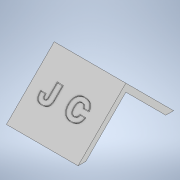
# Autodesk Inventor part: Tablero
Saved by Autodesk Inventor 2022 (Build 260153000, 153)
## iProperties
Created: 2022-08-27
Part Number: Tablero
Material: Generic
Document SubType Name: Modeling
Designer: Wulics
Density: 1 g/cm^3
Appearance: Default
Author: Wulics
Autodesk Inventor part; units mm, degrees
note: some values were not read from the file. Chosen so that the rebuilt part matches the saved one: direction of "Emboss1".
ref_plane "YZ Plane" through (0, 0, 0) normal (1, 0, 0) x (0, 1, 0)
ref_plane "XZ Plane" through (0, 0, 0) normal (0, 1, 0) x (-1, 0, 0)
ref_plane "XY Plane" through (0, 0, 0) normal (0, 0, 1) x (1, 0, 0)
sketch "Sketch1" plane through (0, 0, 0) normal (1, 0, 0) x (0, 1, 0)
  line L0 (0, 0) -> (173.2412, -173.2412)
  line L1 (173.2412, -173.2412) -> (0, -346.4823)
  line L2 (0, -346.4823) -> (0, -318.1981)
  line L3 (0, -318.1981) -> (144.9569, -173.2412)
  line L4 (144.9569, -173.2412) -> (0, -28.2843)
  line L5 (0, -28.2843) -> (0, 0)
  dimension "d0" = 245
  dimension "d1" = 245
  dimension "d2" = 90
  dimension "d3" = 20
  dimension "d4" = 20
  constraints: 12 end point, 2 parallel, 1 collinear, 1 point on line, 1 vertical
  measures "d0" distance of L0.start L0.end
  measures "d1" distance of L0.end L1.end
  measures "d2" angle of L3 L4
  measures "d3" distance between parallel lines of L0 L4
  measures "d4" distance between parallel lines of L1 L3
extrude "Extrusion1" add sketch "Sketch1" along normal blind 260
sketch "Sketch2" plane through (0, 0, 0) normal (0, 0.7071068, 0.7071068) x (1, 0, 0)
  line L0 (37.9204, 161.6588) -> (217.6406, 161.6588) construction
  line L1 (217.6406, 161.6588) -> (217.6406, 17.7751) construction
  line L2 (217.6406, 17.7751) -> (37.9204, 17.7751) construction
  line L3 (37.9204, 17.7751) -> (37.9204, 161.6588) construction
  line L4 (39.9742, 120.0125) -> (59.8275, 120.0125)
  line L5 (59.8275, 120.0125) -> (59.8275, 113.5088)
  spline S0 degree 2 poles (59.8275, 113.5088) (59.8275, 109.173) (62.5088, 105.6359) (65.5895, 105.6359) knots 0 0 0 1 2 2 2
  spline S1 degree 2 poles (65.5895, 105.6359) (68.8413, 105.6359) (71.5227, 109.4583) (71.5227, 115.0492) knots 0 0 0 1 2 2 2
  line L6 (71.5227, 115.0492) -> (71.5227, 159.8332)
  line L7 (71.5227, 159.8332) -> (94.0003, 159.8332)
  line L8 (94.0003, 159.8332) -> (94.0003, 112.7101)
  spline S2 degree 2 poles (94.0003, 112.7101) (94.0003, 100.5585) (79.909, 87.8935) (66.3312, 87.8935) knots 0 0 0 1 2 2 2
  spline S3 degree 2 poles (66.3312, 87.8935) (52.6392, 87.8935) (39.9742, 101.4143) (39.9742, 116.1331) knots 0 0 0 1 2 2 2
  line L9 (39.9742, 116.1331) -> (39.9742, 120.0125)
  line L10 (57.4314, 111.6832) -> (57.4314, 117.7875)
  line L11 (57.4314, 117.7875) -> (42.4844, 117.7875)
  line L12 (42.4844, 117.7875) -> (42.4844, 114.9351)
  spline S4 degree 2 poles (42.4844, 114.9351) (42.4844, 102.213) (54.3507, 90.1184) (66.8446, 90.1184) knots 0 0 0 1 2 2 2
  spline S5 degree 2 poles (66.8446, 90.1184) (79.3385, 90.1184) (91.5471, 102.27) (91.5471, 114.6498) knots 0 0 0 1 2 2 2
  line L13 (91.5471, 114.6498) -> (91.5471, 157.4371)
  line L14 (91.5471, 157.4371) -> (73.9188, 157.4371)
  line L15 (73.9188, 157.4371) -> (73.9188, 113.3377)
  spline S6 degree 2 poles (73.9188, 113.3377) (73.9188, 108.032) (69.8682, 103.411) (65.2472, 103.411) knots 0 0 0 1 2 2 2
  spline S7 degree 2 poles (65.2472, 103.411) (61.539, 103.411) (57.4314, 107.7468) (57.4314, 111.6832) knots 0 0 0 1 2 2 2
  line L16 (184.31, 116.9888) -> (205.5895, 116.9888)
  spline S8 degree 2 poles (205.5895, 116.9888) (204.7338, 103.2399) (187.0483, 87.8935) (172.0443, 87.8935) knots 0 0 0 1 2 2 2
  spline S9 degree 2 poles (172.0443, 87.8935) (155.2146, 87.8935) (135.9318, 107.6327) (135.9318, 124.8047) knots 0 0 0 1 2 2 2
  spline S10 degree 2 poles (135.9318, 124.8047) (135.9318, 141.8625) (155.0435, 161.6588) (171.5308, 161.6588) knots 0 0 0 1 2 2 2
  spline S11 degree 2 poles (171.5308, 161.6588) (186.706, 161.6588) (204.2203, 146.9399) (205.1902, 133.3621) knots 0 0 0 1 2 2 2
  line L17 (205.1902, 133.3621) -> (183.6824, 133.3621)
  spline S12 degree 2 poles (183.6824, 133.3621) (183.226, 138.7248) (177.2358, 144.1445) (171.8161, 144.1445) knots 0 0 0 1 2 2 2
  spline S13 degree 2 poles (171.8161, 144.1445) (165.1983, 144.1445) (158.5805, 134.5031) (158.5805, 124.7476) knots 0 0 0 1 2 2 2
  spline S14 degree 2 poles (158.5805, 124.7476) (158.5805, 115.2203) (165.5977, 105.4077) (172.4436, 105.4077) knots 0 0 0 1 2 2 2
  spline S15 degree 2 poles (172.4436, 105.4077) (177.5781, 105.4077) (183.7965, 111.455) (184.31, 116.9888) knots 0 0 0 1 2 2 2
  line L18 (202.9082, 114.7639) -> (186.4208, 114.7639)
  spline S16 degree 2 poles (186.4208, 114.7639) (185.7362, 109.5153) (178.0345, 103.2399) (172.3295, 103.2399) knots 0 0 0 1 2 2 2
  spline S17 degree 2 poles (172.3295, 103.2399) (164.4567, 103.2399) (156.0704, 114.2505) (156.0704, 124.7476) knots 0 0 0 1 2 2 2
  spline S18 degree 2 poles (156.0704, 124.7476) (156.0704, 135.4729) (164.1714, 146.2553) (172.3295, 146.2553) knots 0 0 0 1 2 2 2
  spline S19 degree 2 poles (172.3295, 146.2553) (177.8633, 146.2553) (185.0516, 140.6645) (185.9074, 135.6441) knots 0 0 0 1 2 2 2
  line L19 (185.9074, 135.6441) -> (202.0524, 135.6441)
  spline S20 degree 2 poles (202.0524, 135.6441) (201.0826, 146.8258) (185.2798, 159.5479) (172.2154, 159.5479) knots 0 0 0 1 2 2 2
  spline S21 degree 2 poles (172.2154, 159.5479) (156.3556, 159.5479) (138.442, 141.1209) (138.442, 124.8047) knots 0 0 0 1 2 2 2
  spline S22 degree 2 poles (138.442, 124.8047) (138.442, 108.4314) (156.2415, 90.1184) (172.2725, 90.1184) knots 0 0 0 1 2 2 2
  spline S23 degree 2 poles (172.2725, 90.1184) (185.5651, 90.1184) (201.596, 103.0117) (202.9082, 114.7639) knots 0 0 0 1 2 2 2
  point P0 (0, 0)
  constraints: 2 other
emboss "Emboss1" sketch "Sketch2" operation cut depth 5 direction (0, -0.7071068, -0.7071068)
body "Solid1"
